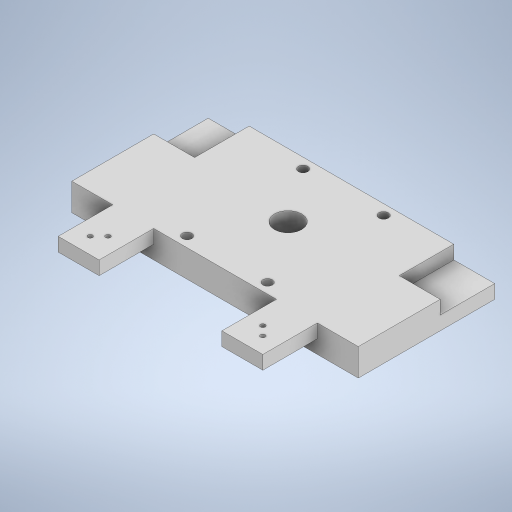
# Autodesk Inventor part: base_mid
Saved by Autodesk Inventor 2023 (Build 270158000, 158)
## iProperties
Created: 2022-10-22
Part Number: base_mid
Material: Genérico
Document SubType Name: Modeling
Designer: inigo
Density: 1 g/cm^3
Appearance: Valor por defecto
Author: inigo
Autodesk Inventor part; units mm, degrees
ref_plane "YZ Plane" through (0, 0, 0) normal (1, 0, 0) x (0, 1, 0)
ref_plane "XZ Plane" through (0, 0, 0) normal (0, 1, 0) x (-1, 0, 0)
ref_plane "XY Plane" through (0, 0, 0) normal (0, 0, 1) x (1, 0, 0)
sketch "Boceto1" plane through (0, 0, 0) normal (0, 1, 0) x (-1, 0, 0)
  line L0 (105, 50) -> (-105, 50)
  line L1 (-105, 50) -> (-105, -50)
  line L2 (-105, -50) -> (105, -50)
  line L3 (105, -50) -> (105, 50)
  line L4 (105, 50) -> (-105, -50) construction
  line L5 (-105, 50) -> (105, -50) construction
  point P0 (0, 0)
  dimension "d0" = 210
  dimension "d1" = 100
  constraints: 12 end point, 2 midpoint, 2 parallel, 1 horizontal, 1 perpendicular
  measures "d0" distance of L2.end L1.end
  measures "d1" distance of L1.end L0.end
extrude "Extrusión1" add sketch "Boceto1" along normal blind 20
sketch "Boceto2" plane through (0, 20, 0) normal (0, 1, 0) x (1, 0, 0)
  circle A0 centre (0, 3.5) radius 10
  circle A1 centre (31, -42.5) radius 3.5
  line L0 (0, 3.5) -> (21.5607, 3.5)
  circle A2 centre (31, 42.5) radius 3.5
  circle A3 centre (-28, 42.5) radius 3.5
  circle A4 centre (-28, -42.5) radius 3.5
  line L1 (105, 50) -> (-105, 50) projected
  point P0 (0, 0)
  dimension "d4" = 7
  dimension "d5" = 7
  dimension "d6" = 7
  dimension "d7" = 39
  dimension "d8" = 46
  dimension "d9" = 59
  dimension "d10" = 46
  dimension "d11" = 39
  dimension "d12" = 59
  dimension "d13" = 7.5
  constraints: 5 centre point, 2 end point, 1 horizontal
  measures "d4" diameter of A1
  measures "d5" diameter of A2
  measures "d6" diameter of A4
  measures "d7" vertical distance of L0.start A3.centre
  measures "d8" vertical distance of L0.start A4.centre
  measures "d9" distance of A4.centre A1.centre
  measures "d10" vertical distance of L0.start A1.centre
  measures "d11" vertical distance of A2.centre L0.start
  measures "d12" distance between centres of A3 A2
  measures "d13" distance from line of L1 A3.centre
extrude "Extrusión2" cut sketch "Boceto2" against normal blind 20
sketch "Boceto3" plane through (0, 20, 0) normal (0, 1, 0) x (1, 0, 0)
  line L0 (-105, -50) -> (105, -50) projected
  line L1 (-45.0001, -10) -> (-45.0001, -50)
  line L2 (-75, -10) -> (-45.0001, -10)
  line L3 (-75, -50) -> (-75, -10)
  line L4 (-65, -50) -> (-75, -50)
  line L5 (-45.0001, -50) -> (-75, -50)
  line L6 (-55, -50.0503) -> (-45.0001, -50)
  line L7 (105, -50) -> (-105, -50)
  line L8 (55, -50.0503) -> (45.0001, -50)
  line L9 (65, -50) -> (75, -50)
  line L10 (-105, -50) -> (105, -50)
  line L11 (0, -50) -> (0, -28.25)
  line L12 (45.0001, -10) -> (45.0001, -50)
  line L13 (45.0001, -50) -> (75, -50)
  line L14 (75, -50) -> (75, -10)
  line L15 (75, -10) -> (45.0001, -10)
  point P0 (0, 0)
  constraints: 30 end point, 6 point on line
extrude "Extrusión3" cut sketch "Boceto3" against normal blind 10
sketch "Boceto4" plane through (-75, 20, 10) normal (0, 0, 1) x (1, 0, 0)
  line L0 (0, -10) -> (0, 0) projected
  line L1 (29.9999, -10) -> (0, -10) projected
  line L2 (0, 0) -> (29.9999, 0)
  line L3 (29.9999, 0) -> (29.9999, -10)
  line L4 (29.9999, -10) -> (0, -10)
  line L5 (0, -10) -> (0, 0)
  line L6 (120.0001, -10) -> (120.0001, 0) projected
  line L7 (150, -10) -> (120.0001, -10) projected
  line L8 (120.0001, 0) -> (150, 0)
  line L9 (150, 0) -> (150, -10)
  line L10 (150, -10) -> (120.0001, -10)
  line L11 (120.0001, -10) -> (120.0001, 0)
  point P0 (75, -20)
  constraints: 16 end point, 4 parallel, 2 horizontal, 2 perpendicular
extrude "Extrusión4" add sketch "Boceto4" along normal blind 80
sketch "Boceto5" plane through (0, 20, 0) normal (0, 1, 0) x (1, 0, 0)
  circle A0 centre (56.75, -71.75) radius 1.75
  line L0 (55, -71.75) -> (55, -49.9497)
  circle A1 centre (63.25, -78.25) radius 1.75
  line L1 (65, -78.25) -> (65, -50)
  line L2 (105, -50) -> (-105, -50)
  line L3 (55, -49.9497) -> (45.0001, -50)
  line L4 (65, -50) -> (75, -50)
  line L5 (45.0001, -50) -> (75, -50)
  line L6 (75, -50) -> (75, -90)
  line L7 (75, -90) -> (45.0001, -90)
  line L8 (45.0001, -90) -> (45.0001, -50)
  line L9 (0, -50) -> (0, -71.75)
  circle A2 centre (-56.75, -71.75) radius 1.75
  line L10 (-55, -71.75) -> (-55, -49.9497)
  circle A3 centre (-63.25, -78.25) radius 1.75
  line L11 (-65, -78.25) -> (-65, -50)
  line L12 (-105, -50) -> (105, -50)
  line L13 (-55, -49.9497) -> (-45.0001, -50)
  line L14 (-65, -50) -> (-75, -50)
  line L15 (-45.0001, -50) -> (-75, -50)
  line L16 (-75, -50) -> (-75, -90)
  line L17 (-75, -90) -> (-45.0001, -90)
  line L18 (-45.0001, -90) -> (-45.0001, -50)
  line L19 (-45.0001, -90) -> (-75, -90) projected
  point P0 (0, 0)
  point P1 (105, 90)
  point P2 (105, 90)
  point P3 (-75, -50)
  point P4 (63.25, -61.75)
  point P5 (56.75, -68.25)
  point P6 (-56.75, -68.25)
  point P7 (-63.25, -61.75)
  dimension "d41" = 3.5
  dimension "d42" = 3.5
  dimension "d33" = 10
  dimension "d34" = 10
  dimension "d35" = 40
  dimension "d36" = 0
  dimension "d37" = 6.5
  dimension "d38" = 6.5
  dimension "d39" = 21.75
  dimension "d40" = 28.25
  dimension "d43" = 11.7499
  dimension "d44" = 11.75
  constraints: 38 end point, 13 symmetric about line, 6 point on line, 6 vertical, 4 horizontal alignment, 2 parallel, 1 horizontal, 1 midpoint, 1 perpendicular, 8 other
  measures "d33" distance of L0.end L5.start
  measures "d34" distance of L4.start L4.end
  measures "d35" distance of L5.end L6.end
  measures "d36" distance between parallel lines of L19 L17
  measures "d37" horizontal distance of point (-63.25, -78.25) point (-56.75, -71.75)
  measures "d38" horizontal distance of point (-63.25, -78.25) point (-56.75, -71.75)
  measures "d39" distance from line of L12 point (-56.75, -71.75)
  measures "d40" distance from line of L2 point (-63.25, -78.25)
  measures "d43" distance from line of L18 point (-56.75, -71.75)
  measures "d44" distance from line of L16 point (-63.25, -78.25)
hole "Agujero1" at (-56.75, 20, 71.75) at (-63.25, 20, 78.25) at (56.75, 20, 71.75) at (63.25, 20, 78.25) direction (0, -1, 0) diameter 3.5 end through all
sketch "Boceto6" plane through (105, 0, -50) normal (0, 0, -1) x (-1, 0, 0)
  line L0 (30, 20) -> (30, 10)
  line L1 (0, 0) -> (0, 20) projected
  line L2 (30, 20) -> (0, 20) projected
  line L3 (0, 20) -> (30, 20)
  line L4 (30, 20) -> (30, 10)
  line L5 (30, 10) -> (0, 10)
  line L6 (0, 10) -> (0, 20)
  line L7 (150.0001, 20) -> (59.9999, 20) projected
  line L8 (105, 20) -> (105, 8.0079)
  line L9 (180, 20) -> (180, 10)
  line L10 (210, 0) -> (210, 20)
  line L11 (180, 20) -> (210, 20)
  line L12 (210, 20) -> (180, 20)
  line L13 (180, 20) -> (180, 10)
  line L14 (180, 10) -> (210, 10)
  line L15 (210, 10) -> (210, 20)
  point P0 (105, 0)
  dimension "d70" = 30
  dimension "d71" = 30
  constraints: 26 end point, 6 symmetric about line, 2 parallel, 1 horizontal, 1 midpoint, 1 perpendicular, 1 vertical
  measures "d70" distance between parallel lines of L1 L0
  measures "d71" distance of L0.end L5.end
extrude "Extrusión6" cut sketch "Boceto6" against normal blind 40
